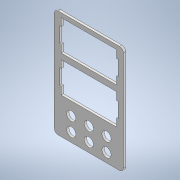
# Autodesk Inventor part: front_case
Saved by Autodesk Inventor 2022.1 (Build 261234020, 234B)
## iProperties
Created: 2022-02-06
Part Number: front_case
Material: Generic
Document SubType Name: Modeling
Designer: kee
Mass: 88.6806 g
Surface Area: 594.98 cm^2
Volume: 88.6806 cm^3
Density: 1 g/cm^3
Appearance: Default
Author: kee
Autodesk Inventor part; units mm, degrees
ref_plane "YZ Plane" through (0, 0, 0) normal (1, 0, 0) x (0, 1, 0)
ref_plane "XZ Plane" through (0, 0, 0) normal (0, 1, 0) x (-1, 0, 0)
ref_plane "XY Plane" through (0, 0, 0) normal (0, 0, 1) x (1, 0, 0)
sketch "Sketch1" plane through (0, 0, 0) normal (0, 0, 1) x (1, 0, 0)
  line L0 (-40, 70) -> (40, 70)
  line L1 (45, 65) -> (45, -65)
  line L2 (40, -70) -> (-40, -70)
  line L3 (-45, -65) -> (-45, 65)
  arc A0 (-40, 70) -> (-45, 65) centre (-40, 65) ccw
  arc A1 (45, 65) -> (40, 70) centre (40, 65) ccw
  arc A2 (-45, -65) -> (-40, -70) centre (-40, -65) ccw
  arc A3 (40, -70) -> (45, -65) centre (40, -65) ccw
  point P0 (0, 0)
  point P1 (-45, 70)
  point P2 (45, -70)
  point P3 (45, 70)
  point P4 (-45, -70)
  point P5 (45, 0)
  dimension "d3" = 90
  dimension "d4" = 45
  dimension "d5" = 140
  dimension "d6" = 70
  dimension "d37" = 5
  constraints: 8 end point, 8 point on circle, 8 point on line, 8 tangent, 4 centre point, 3 equal radius, 2 parallel, 1 horizontal, 1 midpoint, 1 perpendicular
  measures "d3" distance between parallel lines of L1 L3
  measures "d4" distance of point (45, 0) point (0, 0)
  measures "d5" distance between parallel lines of L2 L0
  measures "d6" distance from line of L2 point (0, 0)
  measures "d37" radius of A0
extrude "Extrusion1" add sketch "Sketch1" along normal blind 3
sketch "Sketch2" plane through (0, 0, 3) normal (0, 0, 1) x (1, 0, 0)
  circle A0 centre (-23, -40) radius 6
  circle A1 centre (-23, -58) radius 6
  circle A2 centre (0, -40) radius 6
  circle A3 centre (0, -58) radius 6
  circle A4 centre (23, -40) radius 6
  circle A5 centre (23, -58) radius 6
  line L0 (-40, -70) -> (40, -70) projected
  line L1 (-36, 17) -> (36, 17)
  line L2 (36, 17) -> (36, 7)
  line L3 (36, 7) -> (38, 7)
  line L4 (38, 7) -> (38, -13)
  line L5 (38, -13) -> (36, -13)
  line L6 (36, -13) -> (36, -23)
  line L7 (36, -23) -> (-36, -23)
  line L8 (-36, -23) -> (-36, -13)
  line L9 (-36, -13) -> (-38, -13)
  line L10 (-38, -13) -> (-38, 7)
  line L11 (-38, 7) -> (-36, 7)
  line L12 (-36, 17) -> (-36, 7)
  line L13 (-36, 64.5) -> (36, 64.5)
  line L14 (36, 64.5) -> (36, 54.5)
  line L15 (36, 54.5) -> (38, 54.5)
  line L16 (38, 54.5) -> (38, 34.5)
  line L17 (38, 34.5) -> (36, 34.5)
  line L18 (36, 34.5) -> (36, 24.5)
  line L19 (36, 24.5) -> (-36, 24.5)
  line L20 (-36, 24.5) -> (-36, 34.5)
  line L21 (-36, 34.5) -> (-38, 34.5)
  line L22 (-38, 34.5) -> (-38, 54.5)
  line L23 (-38, 54.5) -> (-36, 54.5)
  line L24 (-36, 64.5) -> (-36, 54.5)
  point P0 (-50, -70)
  point P1 (50, -70)
  point P2 (0, 0)
  point P3 (0, 47.5)
  dimension "d7" = 12
  dimension "d8" = 12
  dimension "d9" = 12
  dimension "d10" = 12
  dimension "d11" = 12
  dimension "d12" = 12
  dimension "d13" = 23
  dimension "d14" = 23
  dimension "d15" = 18
  dimension "d17" = 12
  dimension "d18" = 72
  dimension "d19" = 36
  dimension "d20" = 40
  dimension "d21" = 10
  dimension "d22" = 10
  dimension "d23" = 2
  dimension "d24" = 2
  dimension "d27" = 23
  dimension "d28" = 72
  dimension "d29" = 36
  dimension "d30" = 40
  dimension "d31" = 10
  dimension "d32" = 10
  dimension "d33" = 2
  dimension "d34" = 2
  dimension "d35" = 23
  dimension "d36" = 7.5
  constraints: 48 end point, 14 perpendicular, 14 point on line, 6 centre point, 4 horizontal alignment, 4 vertical alignment, 2 horizontal, 2 vertical
  measures "d7" diameter of A0
  measures "d8" diameter of A1
  measures "d9" diameter of A2
  measures "d10" diameter of A3
  measures "d11" diameter of A4
  measures "d12" diameter of A5
  measures "d13" distance of A2.centre A0.centre
  measures "d14" distance of A4.centre A2.centre
  measures "d15" distance of A5.centre A4.centre
  measures "d17" distance from line of L0 A5.centre
  measures "d18" distance of L1.start L1.end
  measures "d19" distance from line of L2 point (0, 0)
  measures "d20" distance between parallel lines of L7 L1
  measures "d21" distance of L1.end L2.end
  measures "d22" distance of L5.end L6.end
  measures "d23" distance between parallel lines of L4 L6
  measures "d24" distance between parallel lines of L10 L8
  measures "d27" distance from line of L7 point (0, 0)
  measures "d28" distance of L24.start L14.start
  measures "d29" distance from line of L14 point (0, 47.5)
  measures "d30" distance between parallel lines of L19 L13
  measures "d31" distance of L14.start L15.start
  measures "d32" distance of L18.start L19.start
  measures "d33" distance between parallel lines of L16 L18
  measures "d34" distance between parallel lines of L22 L20
  measures "d35" distance from line of L19 point (0, 47.5)
  measures "d36" distance between parallel lines of L1 L19
extrude "Extrusion2" cut sketch "Sketch2" against normal up to next
sketch "Sketch5" plane through (0, 0, 0) normal (0, 0, -1) x (-1, 0, 0)
  circle A0 centre (23, -40) radius 6 projected
  circle A1 centre (0, -58) radius 6 projected
  circle A2 centre (23, -58) radius 6 projected
  line L0 (38, 7) -> (38, -13) projected
  line L1 (38, -13) -> (36, -13) projected
  line L2 (36, -13) -> (36, -23) projected
  line L3 (36, -23) -> (-36, -23) projected
  line L4 (-36, -23) -> (-36, -13) projected
  line L5 (-36, -13) -> (-38, -13) projected
  line L6 (-38, -13) -> (-38, 7) projected
  line L7 (-38, 7) -> (-36, 7) projected
  line L8 (-36, 7) -> (-36, 17) projected
  line L9 (-36, 17) -> (36, 17) projected
  line L10 (36, 17) -> (36, 7) projected
  line L11 (36, 7) -> (38, 7) projected
  circle A3 centre (0, -40) radius 6 projected
  circle A4 centre (-23, -58) radius 6 projected
  circle A5 centre (-23, -40) radius 6 projected
  line L12 (38, 54.5) -> (38, 34.5) projected
  line L13 (38, 34.5) -> (36, 34.5) projected
  line L14 (36, 34.5) -> (36, 24.5) projected
  line L15 (36, 24.5) -> (-36, 24.5) projected
  line L16 (-36, 24.5) -> (-36, 34.5) projected
  line L17 (-36, 34.5) -> (-38, 34.5) projected
  line L18 (-38, 34.5) -> (-38, 54.5) projected
  line L19 (-38, 54.5) -> (-36, 54.5) projected
  line L20 (-36, 54.5) -> (-36, 64.5) projected
  line L21 (-36, 64.5) -> (36, 64.5) projected
  line L22 (36, 64.5) -> (36, 54.5) projected
  line L23 (36, 54.5) -> (38, 54.5) projected
  line L24 (40, -70) -> (-40, -70) projected
  arc A6 (40, -70) -> (45, -65) centre (40, -65) ccw projected
  line L25 (45, 65) -> (45, -65) projected
  arc A7 (45, 65) -> (40, 70) centre (40, 65) ccw projected
  line L26 (-40, 70) -> (40, 70) projected
  arc A8 (-40, 70) -> (-45, 65) centre (-40, 65) ccw projected
  line L27 (-45, -65) -> (-45, 65) projected
  arc A9 (-45, -65) -> (-40, -70) centre (-40, -65) ccw projected
  arc A10 (42, 65) -> (40, 67) centre (40, 65) ccw
  line L28 (42, 65) -> (42, -65)
  arc A11 (40, -67) -> (42, -65) centre (40, -65) ccw
  line L29 (40, -67) -> (-40, -67)
  arc A12 (-42, -65) -> (-40, -67) centre (-40, -65) ccw
  line L30 (-42, -65) -> (-42, 65)
  arc A13 (-40, 67) -> (-42, 65) centre (-40, 65) ccw
  line L31 (-40, 67) -> (40, 67)
  line L32 (-40, 70) -> (40, 70)
  arc A14 (45, 65) -> (40, 70) centre (40, 65) ccw
  line L33 (45, 65) -> (45, -65)
  arc A15 (40, -70) -> (45, -65) centre (40, -65) ccw
  line L34 (40, -70) -> (-40, -70)
  arc A16 (-45, -65) -> (-40, -70) centre (-40, -65) ccw
  line L35 (-45, -65) -> (-45, 65)
  arc A17 (-40, 70) -> (-45, 65) centre (-40, 65) ccw
  arc A18 (-40, 62) -> (-37, 65) centre (-40, 65) ccw
  line L36 (-37, 65) -> (-37, 67)
  line L37 (-40, 62) -> (-42, 62)
  line L38 (-116.3396, 0) -> (109.1655, 0) construction
  line L39 (0, 86.6309) -> (0, -88.1774) construction
  arc A19 (37, 65) -> (40, 62) centre (40, 65) ccw
  line L40 (37, 65) -> (37, 67)
  line L41 (40, 62) -> (42, 62)
  arc A20 (-37, -65) -> (-40, -62) centre (-40, -65) ccw
  line L42 (-37, -65) -> (-37, -67)
  line L43 (-40, -62) -> (-42, -62)
  line L44 (37, -65) -> (37, -67)
  arc A21 (40, -62) -> (37, -65) centre (40, -65) ccw
  line L45 (40, -62) -> (42, -62)
  point P0 (0, 0)
  dimension "d38" = 3
  dimension "d39" = 3
  constraints: 36 end point, 24 point on circle, 15 symmetric about line, 12 centre point, 7 tangent, 5 coincident, 4 perpendicular, 4 point on line, 2 horizontal, 1 vertical, 10 other
  measures "d38" distance between parallel lines of L26 L31
  measures "d39" radius of A18
extrude "Extrusion3" add sketch "Sketch5" along normal blind 50 contours L24 A9 L27 A8 L26 A7 L25 A6 | L28 L41 A19 L40 L31 A10 | L28 A11 L29 L44 A21 L45 | L36 A18 L37 L30 A13 L31 | L29 A12 L30 L43 A20 L42
equation "\"d4\" = 0.5 * d3"
equation "\"d6\" = 0.5 * d5"
equation "\"d14\" = d13"
equation "\"d19\" = 0.5 * d18"
equation "\"d29\" = 0.5 * d28"
body "Solid1"
